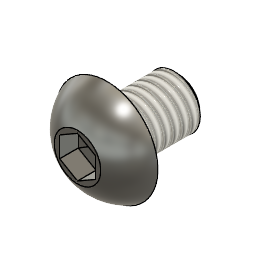
fpv frame (Autodesk Fusion 360 archive; units mm, degrees)
design "Broached Hexagon Socket Button Head Cap Screw ANSI B18.3.4M - M3 x 0.5 x 4 Steel Grade 2 Plain"
description: Broached Hexagon Socket Button Head Cap Screw ANSI B18.3.4M - M3 x 0.5 x 4
part number: BHSBHCS ANSI B18.3.4M - M3 x 0.5 x 4 Steel Grade 2 Plain
Autodesk Fusion 360 part; units mm, degrees
sketch "Sketch1" plane through (0, 0, 0) normal (0, 1, 0) x (1, 0, 0)
  line L0 (-1.5, 0) -> (-1.5, 4)
  line L1 (-1.5, 4) -> (0, 4)
  line L2 (0, 4) -> (0, -1.65)
  line L3 (-1.5, 0) -> (-2.85, 0)
  line L4 (0, -1.65) -> (-1.3, -1.65)
  arc A0 (-2.85, 0) -> (-1.3, -1.65) centre (0, 1.1242) ccw
  dimension "d9" = 3
  dimension "d66" = 5.7
  dimension "d98" = 2.6
  dimension "d105" = 1.65
  dimension "d106" = 4
  constraint perpendicular L0 L1
  constraint perpendicular L0 L3
  constraint coincident origin L3
  constraint vertical L0
  constraint vertical L2
  constraint coincident origin L2
  constraint perpendicular L2 L4
  constraint coincident L2 A0.centre
  measures "d105" distance of L3 L4
  measures "d106" distance of origin L1
revolve "Revolve1" add sketch "Sketch1" angle 360 about axis through (0, 0, -4) along (0, 0, 1)
ref_plane "WorkPlane1" through (0, 0, 1.65) normal (0, 0, 1) x (1, 0, 0)
sketch "Sketch6" plane through (0, 0, 1.65) normal (0, 0, 1) x (1, 0, 0)
  line L0 (0, -1.1547) -> (1, -0.5774)
  line L1 (1, -0.5774) -> (1, 0.5774)
  line L2 (1, 0.5774) -> (0, 1.1547)
  line L3 (0, 1.1547) -> (-1, 0.5774)
  line L4 (-1, 0.5774) -> (-1, -0.5774)
  line L5 (-1, -0.5774) -> (0, -1.1547)
  dimension "d117" = 2
  constraint vertical L1
  measures "d117" distance of L1 L4
extrude "Extrude1" cut sketch "Sketch6" against normal blind 1.04
extrude "Extrude2" cut 1 faces at (-0.3333, -0.1925, 0.61) along direction (0, 0, -1) blind 1.04 draft -85
fillet "Fillet5" radius 0.1 1 edges at (-1.3985, 0.5424, 0)
thread "Thread5" "ANSI Metric M Profile 3.0 M3x0.5 M3x0.5 4g6g" major diameter 2.927 minor diameter 2.369 pitch 0.5 angle 60 resizes the face on face at (-1.4981, 0.0748, -2.7) from (0, 0, -1) to (0, 0, -4)
sketch "Sketch5" plane through (0, 0, 0) normal (0, 1, 0) x (1, 0, 0)
  line L0 (0, 4) -> (0, -1.65)
  line L1 (0, 4) -> (-1.53, 4)
  line L2 (-1.53, 4) -> (-1.53, 3.6933)
  line L3 (-1.53, 3.6933) -> (-1.1933, 4)
  dimension "d108" = 0.3067
  dimension "d109" = 1.1933
  dimension "d110" = 1.53
  constraint coincident L0.start L1.start
  constraint perpendicular L1 L2
  constraint coincident L1 L3.end
  measures "d108" distance of L1 L2.end
  measures "d109" distance of L0 L3.end
  measures "d110" distance of L0 L2
revolve "Revolve2" cut sketch "Sketch5" angle 360 about axis through (0, 0, -4) along (0, 0, 1)
equation "d9 = adsk_nomdia"
equation "adsk_nomlen = 4.00 mm"
equation "adsk_headh = 1.65 mm"
equation "adsk_headdia = 5.70 mm"
equation "adsk_nomdia = 3.00 mm"
equation "adsk_philwidth = 2.00 mm"
equation "d31 = -adsk_phildepth"
equation "adsk_phildepth = 1.04 mm"
equation "d66 = adsk_headdia"
equation "d71 = adsk_headh"
equation "d76 = -adsk_phildepth"
equation "adsk_thrlen = 3.00 mm"
equation "adsk_endpointdia = 2.38655 mm"
equation "adsk_startlen = 0.306725 mm"
equation "d98 = adsk_philwidth * 1.3"
equation "adsk_midfillet = 0.10 mm"
equation "d104 = adsk_midfillet"
equation "d105 = adsk_headh"
equation "d106 = adsk_nomlen"
equation "d108 = adsk_startlen"
equation "d109 = adsk_endpointdia / 2"
equation "d110 = adsk_nomdia * 0.51"
equation "d116 = min(adsk_thrlen; adsk_nomlen - adsk_midfillet - 0.001 mm)"
equation "d117 = adsk_philwidth"

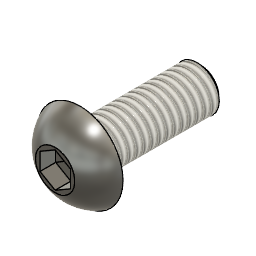
design "Button Head Screw BS 4168-6 - M3 x 8 Steel 4.6 Plain"
description: Button Head Screw BS 4168-6 - M3 x 8
part number: HSBHS BS 4168-6 - M3 x 8 Steel 4.6 Plain
Autodesk Fusion 360 part; units mm, degrees
sketch "Sketch1" plane through (0, 0, 0) normal (0, 1, 0) x (1, 0, 0)
  line L0 (-1.5, 0) -> (-1.5, 8)
  line L1 (-1.5, 8) -> (0, 8)
  line L2 (0, 8) -> (0, -1.65)
  line L3 (-1.5, 0) -> (-2.85, 0)
  line L4 (0, -1.65) -> (-1.3, -1.65)
  arc A0 (-2.85, 0) -> (-1.3, -1.65) centre (0, 1.1242) ccw
  dimension "d9" = 3
  dimension "d66" = 5.7
  dimension "d98" = 2.6
  dimension "d105" = 1.65
  dimension "d106" = 8
  constraint perpendicular L0 L1
  constraint perpendicular L0 L3
  constraint coincident origin L3
  constraint vertical L0
  constraint vertical L2
  constraint coincident origin L2
  constraint perpendicular L2 L4
  constraint coincident L2 A0.centre
  measures "d105" distance of L3 L4
  measures "d106" distance of origin L1
revolve "Revolve1" add sketch "Sketch1" angle 360 about axis through (0, 0, -8) along (0, 0, 1)
ref_plane "WorkPlane1" through (0, 0, 1.65) normal (0, 0, 1) x (1, 0, 0)
sketch "Sketch6" plane through (0, 0, 1.65) normal (0, 0, 1) x (1, 0, 0)
  line L0 (0, -1.1547) -> (1, -0.5774)
  line L1 (1, -0.5774) -> (1, 0.5774)
  line L2 (1, 0.5774) -> (0, 1.1547)
  line L3 (0, 1.1547) -> (-1, 0.5774)
  line L4 (-1, 0.5774) -> (-1, -0.5774)
  line L5 (-1, -0.5774) -> (0, -1.1547)
  dimension "d117" = 2
  constraint vertical L1
  measures "d117" distance of L1 L4
extrude "Extrude1" cut sketch "Sketch6" against normal blind 1.04
extrude "Extrude2" cut 1 faces at (-0.3333, -0.1925, 0.61) along direction (0, 0, -1) blind 1.04 draft -85
fillet "Fillet5" radius 0.1 1 edges at (-1.3985, 0.5424, 0)
thread "Thread5" "ISO Metric profile 3.0 M3x0.5 M3x0.5 6g" major diameter 2.927 minor diameter 2.3555 pitch 0.5 angle 60 resizes the face on face at (-1.4925, 0.1494, -5.3667) from (0, 0, -1) to (0, 0, -8)
sketch "Sketch5" plane through (0, 0, 0) normal (0, 1, 0) x (1, 0, 0)
  line L0 (0, 8) -> (0, -1.65)
  line L1 (0, 8) -> (-1.53, 8)
  line L2 (-1.53, 8) -> (-1.53, 7.6933)
  line L3 (-1.53, 7.6933) -> (-1.1933, 8)
  dimension "d108" = 0.3067
  dimension "d109" = 1.1933
  dimension "d110" = 1.53
  constraint coincident L0.start L1.start
  constraint perpendicular L1 L2
  constraint coincident L1 L3.end
  measures "d108" distance of L1 L2.end
  measures "d109" distance of L0 L3.end
  measures "d110" distance of L0 L2
revolve "Revolve2" cut sketch "Sketch5" angle 360 about axis through (0, 0, -8) along (0, 0, 1)
equation "d9 = adsk_nomdia"
equation "adsk_nomlen = 8.00 mm"
equation "adsk_headh = 1.65 mm"
equation "adsk_headdia = 5.70 mm"
equation "adsk_nomdia = 3.00 mm"
equation "adsk_philwidth = 2.00 mm"
equation "d31 = -adsk_phildepth"
equation "adsk_phildepth = 1.04 mm"
equation "d66 = adsk_headdia"
equation "d71 = adsk_headh"
equation "d76 = -adsk_phildepth"
equation "adsk_thrlen = 7.00 mm"
equation "adsk_endpointdia = 2.38655 mm"
equation "adsk_startlen = 0.306725 mm"
equation "d98 = adsk_philwidth * 1.3"
equation "adsk_midfillet = 0.10 mm"
equation "d104 = adsk_midfillet"
equation "d105 = adsk_headh"
equation "d106 = adsk_nomlen"
equation "d108 = adsk_startlen"
equation "d109 = adsk_endpointdia / 2"
equation "d110 = adsk_nomdia * 0.51"
equation "d116 = min(adsk_thrlen; adsk_nomlen - adsk_midfillet - 0.001 mm)"
equation "d117 = adsk_philwidth"

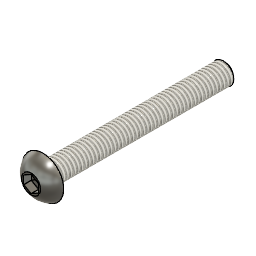
design "Broached Hexagon Socket Button Head Cap Screw ANSI B18.3.4M - M3 x 0.5 x 25 Steel Grade 2 Plain"
description: Broached Hexagon Socket Button Head Cap Screw ANSI B18.3.4M - M3 x 0.5 x 25
part number: BHSBHCS ANSI B18.3.4M - M3 x 0.5 x 25 Steel Grade 2 Plain
Autodesk Fusion 360 part; units mm, degrees
sketch "Sketch1" plane through (0, 0, 0) normal (0, 1, 0) x (1, 0, 0)
  line L0 (-1.5, 0) -> (-1.5, 25)
  line L1 (-1.5, 25) -> (0, 25)
  line L2 (0, 25) -> (0, -1.65)
  line L3 (-1.5, 0) -> (-2.85, 0)
  line L4 (0, -1.65) -> (-1.3, -1.65)
  arc A0 (-2.85, 0) -> (-1.3, -1.65) centre (0, 1.1242) ccw
  dimension "d9" = 3
  dimension "d66" = 5.7
  dimension "d98" = 2.6
  dimension "d105" = 1.65
  dimension "d106" = 25
  constraint perpendicular L0 L1
  constraint perpendicular L0 L3
  constraint coincident origin L3
  constraint vertical L0
  constraint vertical L2
  constraint coincident origin L2
  constraint perpendicular L2 L4
  constraint coincident L2 A0.centre
  measures "d105" distance of L3 L4
  measures "d106" distance of origin L1
revolve "Revolve1" add sketch "Sketch1" angle 360 about axis through (0, 0, -25) along (0, 0, 1)
ref_plane "WorkPlane1" through (0, 0, 1.65) normal (0, 0, 1) x (1, 0, 0)
sketch "Sketch6" plane through (0, 0, 1.65) normal (0, 0, 1) x (1, 0, 0)
  line L0 (0, -1.1547) -> (1, -0.5774)
  line L1 (1, -0.5774) -> (1, 0.5774)
  line L2 (1, 0.5774) -> (0, 1.1547)
  line L3 (0, 1.1547) -> (-1, 0.5774)
  line L4 (-1, 0.5774) -> (-1, -0.5774)
  line L5 (-1, -0.5774) -> (0, -1.1547)
  dimension "d117" = 2
  constraint vertical L1
  measures "d117" distance of L1 L4
extrude "Extrude1" cut sketch "Sketch6" against normal blind 1.04
extrude "Extrude2" cut 1 faces at (-0.3333, -0.1925, 0.61) along direction (0, 0, -1) blind 1.04 draft -85
fillet "Fillet5" radius 0.1 1 edges at (-1.3985, 0.5424, 0)
thread "Thread5" "ANSI Metric M Profile 3.0 M3x0.5 M3x0.5 4g6g" major diameter 2.927 minor diameter 2.369 pitch 0.5 angle 60 resizes the face on face at (-1.4925, 0.1494, -16.7) from (0, 0, -1) to (0, 0, -25)
sketch "Sketch5" plane through (0, 0, 0) normal (0, 1, 0) x (1, 0, 0)
  line L0 (0, 25) -> (0, -1.65)
  line L1 (0, 25) -> (-1.53, 25)
  line L2 (-1.53, 25) -> (-1.53, 24.6933)
  line L3 (-1.53, 24.6933) -> (-1.1933, 25)
  dimension "d108" = 0.3067
  dimension "d109" = 1.1933
  dimension "d110" = 1.53
  constraint coincident L0.start L1.start
  constraint perpendicular L1 L2
  constraint coincident L1 L3.end
  measures "d108" distance of L1 L2.end
  measures "d109" distance of L0 L3.end
  measures "d110" distance of L0 L2
revolve "Revolve2" cut sketch "Sketch5" angle 360 about axis through (0, 0, -25) along (0, 0, 1)
equation "d9 = adsk_nomdia"
equation "adsk_nomlen = 25.00 mm"
equation "adsk_headh = 1.65 mm"
equation "adsk_headdia = 5.70 mm"
equation "adsk_nomdia = 3.00 mm"
equation "adsk_philwidth = 2.00 mm"
equation "d31 = -adsk_phildepth"
equation "adsk_phildepth = 1.04 mm"
equation "d66 = adsk_headdia"
equation "d71 = adsk_headh"
equation "d76 = -adsk_phildepth"
equation "adsk_thrlen = 24.00 mm"
equation "adsk_endpointdia = 2.38655 mm"
equation "adsk_startlen = 0.306725 mm"
equation "d98 = adsk_philwidth * 1.3"
equation "adsk_midfillet = 0.10 mm"
equation "d104 = adsk_midfillet"
equation "d105 = adsk_headh"
equation "d106 = adsk_nomlen"
equation "d108 = adsk_startlen"
equation "d109 = adsk_endpointdia / 2"
equation "d110 = adsk_nomdia * 0.51"
equation "d116 = min(adsk_thrlen; adsk_nomlen - adsk_midfillet - 0.001 mm)"
equation "d117 = adsk_philwidth"
